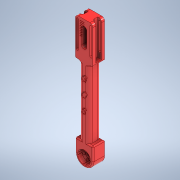
# Autodesk Inventor part: Eslabon1
Saved by Autodesk Inventor 2021 (Build 250183000, 183)
## iProperties
Created: 2022-10-26
Part Number: Eslabon1
Material: Generic
Document SubType Name: Modeling
Designer: USUARIO
Density: 1 g/cm^3
Appearance: Light Red
Mass: 84.0555 g
Surface Area: 248.63 cm^2
Volume: 84.0555 cm^3
Author: USUARIO
Autodesk Inventor part; units mm, degrees
ref_plane "YZ Plane" through (0, 0, 0) normal (1, 0, 0) x (0, 1, 0)
ref_plane "XZ Plane" through (0, 0, 0) normal (0, 1, 0) x (-1, 0, 0)
ref_plane "XY Plane" through (0, 0, 0) normal (0, 0, 1) x (1, 0, 0)
sketch "Sketch1" plane through (0, 0, 0) normal (0, 0, 1) x (1, 0, 0)
  line L0 (0, 0) -> (0, 190) construction
  line L1 (15, 0) -> (15, 190)
  line L2 (-15, 190) -> (-15, 0)
  arc A0 (-15, 0) -> (15, 0) centre (0, 0) ccw
  arc A1 (15, 190) -> (-15, 190) centre (0, 190) ccw
  line L3 (-15, 175) -> (15, 175)
  line L4 (15, 175) -> (15, 200)
  line L5 (10, 205) -> (-10, 205)
  line L6 (-15, 200) -> (-15, 175)
  line L7 (-15, 175) -> (15, 205) construction
  line L8 (15, 175) -> (-15, 205) construction
  arc A2 (-10, 205) -> (-15, 200) centre (-10, 200) ccw
  arc A3 (15, 200) -> (10, 205) centre (10, 200) ccw
  point P0 (0, 95)
  point P1 (0, 205)
  dimension "d0" = 190
  dimension "d1" = 30
  dimension "d48" = 5
  dimension "d49" = 30
  dimension "d50" = 30
  constraints: 20 end point, 8 point on circle, 8 tangent, 4 centre point, 4 point on line, 3 midpoint, 3 parallel, 1 equal radius, 1 horizontal, 1 perpendicular, 1 vertical
  measures "d0" distance of L0.start L0.end
  measures "d1" diameter of A1
  measures "d48" radius of A2
  measures "d49" distance between parallel lines of L6 L4
  measures "d50" distance between parallel lines of L3 L5
extrude "Extrusion1" add sketch "Sketch1" along normal blind 20
sketch "Sketch2" plane through (0, 0, 20) normal (0, 0, 1) x (1, 0, 0)
  arc A0 (15, 185) -> (-15, 185) centre (0, 185) ccw projected
  arc A1 (-15, 0) -> (15, 0) centre (0, 0) ccw projected
  circle A2 centre (0, 0) radius 11
  dimension "d4" = 22
  constraints: 1 centre point, 1 coincident
  measures "d4" diameter of A2
extrude "Extrusion2" cut sketch "Sketch2" against normal blind 7
sketch "Sketch3" plane through (0, 0, 0) normal (0, 0, -1) x (-1, 0, 0)
  circle A0 centre (0, 0) radius 11 projected
  circle A1 centre (0, 0) radius 11
  circle A2 centre (0, 0) radius 2
  circle A3 centre (0, 0) radius 8 construction
  arc A4 (15, 185) -> (-15, 185) centre (0, 185) ccw construction
  circle A5 centre (0, 8) radius 1.5
  line L0 (0, 0) -> (0, 12.8172) construction
  circle A6 centre (-8, 0) radius 1.5
  circle A7 centre (0, -8) radius 1.5
  circle A8 centre (8, 0) radius 1.5
  circle A9 centre (0, 0) radius 5
  dimension "d9" = 16
  dimension "d7" = 22
  dimension "d8" = 4
  dimension "d10" = 3
  dimension "d13" = 360
  dimension "d15" = 10
  constraints: 7 centre point, 4 coincident, 2 end point, 1 point on line, 1 vertical, 1 vertical alignment, 11 other
  measures "d7" diameter of A1
  measures "d8" diameter of A2
  measures "d10" diameter of A5
  measures "d15" diameter of A9
extrude "Extrusion4" cut sketch "Sketch3" against normal through all contours A5 | A6 | A7 | A8
sketch "Sketch4" plane through (0, 0, 13) normal (0, 0, 1) x (1, 0, 0)
  circle A0 centre (-8, 0) radius 1.5 projected
  circle A1 centre (0, 0) radius 2 construction
  circle A2 centre (0, 0) radius 8 construction
  line L0 (-5, 1.7321) -> (-5, -1.7321)
  line L1 (-5, -1.7321) -> (-8, -3.4641)
  line L2 (-8, -3.4641) -> (-11, -1.7321)
  line L3 (-11, -1.7321) -> (-11, 1.7321)
  line L4 (-11, 1.7321) -> (-8, 3.4641)
  line L5 (-8, 3.4641) -> (-5, 1.7321)
  line L6 (-3.4641, -8) -> (-1.7321, -5)
  line L7 (-1.7321, -5) -> (1.7321, -5)
  line L8 (1.7321, -5) -> (3.4641, -8)
  line L9 (3.4641, -8) -> (1.7321, -11)
  line L10 (1.7321, -11) -> (-1.7321, -11)
  line L11 (-1.7321, -11) -> (-3.4641, -8)
  line L12 (8, -3.4641) -> (5, -1.7321)
  line L13 (5, -1.7321) -> (5, 1.7321)
  line L14 (5, 1.7321) -> (8, 3.4641)
  line L15 (8, 3.4641) -> (11, 1.7321)
  line L16 (11, 1.7321) -> (11, -1.7321)
  line L17 (11, -1.7321) -> (8, -3.4641)
  line L18 (3.4641, 8) -> (1.7321, 5)
  line L19 (1.7321, 5) -> (-1.7321, 5)
  line L20 (-1.7321, 5) -> (-3.4641, 8)
  line L21 (-3.4641, 8) -> (-1.7321, 11)
  line L22 (-1.7321, 11) -> (1.7321, 11)
  line L23 (1.7321, 11) -> (3.4641, 8)
  dimension "d20" = 6
  dimension "d23" = 360
  constraints: 48 end point, 3 coincident, 1 horizontal alignment, 1 vertical, 64 other
  measures "d20" distance between parallel lines of L3 L0
extrude "Extrusion5" cut sketch "Sketch4" along normal blind 8.175 and the other way blind 3.5
extrude "Extrusion6" cut sketch "Sketch3" against normal blind 2 contours A0 | A2 | A9
extrude "Extrusion7" cut sketch "Sketch3" against normal through all contours A2
sketch "Sketch5" plane through (0, 0, 13) normal (0, 0, 1) x (1, 0, 0)
  circle A0 centre (0, 0) radius 2 projected
  circle A1 centre (0, 0) radius 4.5
  dimension "d33" = 9
  constraints: 1 centre point, 1 coincident
  measures "d33" diameter of A1
extrude "Extrusion8" cut sketch "Sketch5" against normal blind 3
sketch "Sketch9" plane through (0, 0, 20) normal (0, 0, 1) x (1, 0, 0)
  line L0 (-15, 200) -> (-15, 0) projected
  arc A0 (-15, 0) -> (15, 0) centre (0, 0) ccw projected
  line L1 (15, 0) -> (15, 200) projected
  arc A1 (15, 200) -> (10, 205) centre (10, 200) ccw projected
  line L2 (10, 205) -> (-10, 205) projected
  arc A2 (-10, 205) -> (-15, 200) centre (-10, 200) ccw projected
  line L3 (10.8485, 1.8195) -> (11, 1.7321) projected
  line L4 (11, 1.7321) -> (11, -1.7321) projected
  line L5 (11, -1.7321) -> (10.8485, -1.8195) projected
  arc A3 (1.8195, -10.8485) -> (10.8485, -1.8195) centre (0, 0) ccw projected
  line L6 (1.8195, -10.8485) -> (1.7321, -11) projected
  line L7 (1.7321, -11) -> (-1.7321, -11) projected
  line L8 (-1.7321, -11) -> (-1.8195, -10.8485) projected
  arc A4 (-10.8485, -1.8195) -> (-1.8195, -10.8485) centre (0, 0) ccw projected
  line L9 (-10.8485, -1.8195) -> (-11, -1.7321) projected
  line L10 (-11, -1.7321) -> (-11, 1.7321) projected
  line L11 (-11, 1.7321) -> (-10.8485, 1.8195) projected
  arc A5 (-1.8195, 10.8485) -> (-10.8485, 1.8195) centre (0, 0) ccw projected
  line L12 (-1.8195, 10.8485) -> (-1.7321, 11) projected
  line L13 (-1.7321, 11) -> (1.7321, 11) projected
  line L14 (1.7321, 11) -> (1.8195, 10.8485) projected
  arc A6 (10.8485, 1.8195) -> (1.8195, 10.8485) centre (0, 0) ccw projected
  line L15 (10, 205) -> (-10, 205) projected
  circle A7 centre (0, 0) radius 2 projected
  line L16 (0, 205) -> (0, 0) construction
  line L17 (0, 190) -> (0, 165) construction
  line L18 (-4.5, 190) -> (-4.5, 165)
  line L19 (4.5, 165) -> (4.5, 190)
  arc A8 (4.5, 190) -> (-4.5, 190) centre (0, 190) ccw
  arc A9 (-4.5, 165) -> (4.5, 165) centre (0, 165) ccw
  point P0 (0, 177.5)
  dimension "d51" = 25
  dimension "d52" = 9
  dimension "d53" = 190
  constraints: 10 end point, 4 point on circle, 4 tangent, 2 centre point, 2 midpoint, 2 point on line, 1 parallel, 1 vertical
  measures "d51" distance of L17.start L17.end
  measures "d52" diameter of A9
  measures "d53" distance of point (0, 0) L17.start
extrude "Extrusion11" cut sketch "Sketch9" against normal through all contours A8 L19 A9 L18
sketch "Sketch10" plane through (-10, 205, 0) normal (0, 1, 0) x (1, 0, 0)
  line L0 (14.5, -20) -> (5.5, -20) projected
  line L1 (5.5, -20) -> (14.5, -20) projected
  line L2 (-5, -20) -> (25, -20) projected
  line L3 (25, -20) -> (20, -20) projected
  line L4 (20, -20) -> (0, -20) projected
  line L5 (0, -20) -> (-5, -20) projected
  line L6 (20.8485, -20) -> (21, -20) projected
  line L7 (21, -20) -> (20.8485, -20) projected
  line L8 (20.8485, -20) -> (11.8195, -20) projected
  line L9 (11.8195, -20) -> (11.7321, -20) projected
  line L10 (11.7321, -20) -> (8.2679, -20) projected
  line L11 (8.2679, -20) -> (8.1805, -20) projected
  line L12 (8.1805, -20) -> (-0.8485, -20) projected
  line L13 (-0.8485, -20) -> (-1, -20) projected
  line L14 (-1, -20) -> (-0.8485, -20) projected
  line L15 (-0.8485, -20) -> (8.1805, -20) projected
  line L16 (8.1805, -20) -> (8.2679, -20) projected
  line L17 (8.2679, -20) -> (11.7321, -20) projected
  line L18 (11.7321, -20) -> (11.8195, -20) projected
  line L19 (11.8195, -20) -> (20.8485, -20) projected
  line L20 (25, 0) -> (25, -20) projected
  line L21 (25, 0) -> (25, -20) projected
  line L22 (14.5, 0) -> (5.5, 0) projected
  line L23 (5.5, 0) -> (14.5, 0) projected
  line L24 (-1, 0) -> (21, 0) projected
  line L25 (0, 0) -> (-5, 0) projected
  line L26 (20, 0) -> (0, 0) projected
  line L27 (25, 0) -> (20, 0) projected
  line L28 (-5, 0) -> (25, 0) projected
  line L29 (-5, 0) -> (-5, -20) projected
  line L30 (-5, 0) -> (-5, -20) projected
  line L31 (-5, 0) -> (-5, -20) projected
  line L32 (-5, -5) -> (2, -5)
  line L33 (2, -5) -> (2, -15)
  line L34 (2, -15) -> (-5, -15)
  line L35 (-5, -15) -> (-5, -5)
  line L36 (10, 0) -> (10, -20)
  line L37 (-5, -20) -> (25, -20) projected
  line L38 (25, -5) -> (18, -5)
  line L39 (18, -5) -> (18, -15)
  line L40 (18, -15) -> (25, -15)
  line L41 (25, -15) -> (25, -5)
  point P0 (-5, -15)
  dimension "d56" = 5
  dimension "d57" = 5
  dimension "d58" = 7
  constraints: 18 end point, 4 symmetric about line, 2 parallel, 1 horizontal, 1 perpendicular, 4 other
  measures "d56" distance between parallel lines of L28 L32
  measures "d57" distance between parallel lines of L2 L34
  measures "d58" distance of L33.end L34.end
extrude "Extrusion12" cut sketch "Sketch10" against normal blind 60 contours L40 L39 L38 L20 | L32 L33 L34 L29
sketch "Sketch11" plane through (0, 0, 0) normal (0, 0, -1) x (-1, 0, 0)
  arc A0 (-10, 205) -> (-15, 200) centre (-10, 200) ccw projected
  line L0 (-15, 145) -> (-15, 200) projected
  line L1 (-15, 145) -> (-8, 145) projected
  line L2 (-8, 205) -> (-8, 145) projected
  line L3 (-10, 205) -> (-8, 205) projected
  arc A1 (15, 200) -> (10, 205) centre (10, 200) ccw projected
  line L4 (8, 205) -> (10, 205) projected
  line L5 (8, 205) -> (8, 145) projected
  line L6 (8, 145) -> (15, 145) projected
  line L7 (15, 200) -> (15, 145) projected
  line L8 (-11.5, 145) -> (-11.5, 208.2052) construction
  line L9 (-11.5, 200) -> (-11.5, 155) construction
  line L10 (-13.2, 200) -> (-13.2, 155)
  line L11 (-9.8, 155) -> (-9.8, 200)
  arc A2 (-9.8, 200) -> (-13.2, 200) centre (-11.5, 200) ccw
  arc A3 (-13.2, 155) -> (-9.8, 155) centre (-11.5, 155) ccw
  arc A4 (-4.5, 165) -> (4.5, 165) centre (0, 165) ccw projected
  line L12 (4.5, 190) -> (4.5, 165) projected
  line L13 (-4.5, 165) -> (-4.5, 190) construction
  line L14 (-4.5, 177.5) -> (-11.5, 177.5) construction
  line L15 (-10, 205) -> (10, 205) projected
  line L16 (0, 205) -> (0, 150.8166) construction
  line L17 (13.2, 200) -> (13.2, 155)
  line L18 (9.8, 155) -> (9.8, 200)
  arc A5 (13.2, 200) -> (9.8, 200) centre (11.5, 200) ccw
  arc A6 (9.8, 155) -> (13.2, 155) centre (11.5, 155) ccw
  point P0 (0, 0)
  dimension "d61" = 3.4
  dimension "d62" = 45
  dimension "d73" = 23
  constraints: 18 end point, 8 point on circle, 6 symmetric about line, 4 centre point, 4 midpoint, 4 tangent, 2 point on line, 2 vertical, 1 horizontal, 1 parallel, 2 other
  measures "d61" diameter of A3
  measures "d62" distance of L10.start L10.end
  measures "d73" distance of A5.centre L9.start
extrude "Extrusion13" cut sketch "Sketch11" against normal through all contours A2 L11 A3 L10 | L17 A6 L18 A5
fillet "Fillet1" radius 4 2 edges at (8, 175, 15) (-8, 175, 15)
sketch "Sketch12" plane through (0, 0, 20) normal (0, 0, 1) x (1, 0, 0)
  line L0 (-18.3068, 122.2397) -> (15.3464, 122.2397) construction
  line L1 (15.3464, 122.2397) -> (15.3464, 18.2543) construction
  line L2 (15.3464, 18.2543) -> (-18.3068, 18.2543) construction
  line L3 (-18.3068, 18.2543) -> (-18.3068, 122.2397) construction
  line L4 (4.9339, 119.3269) -> (3.4605, 118.9967)
  spline S0 degree 2 poles (3.4605, 118.9967) (3.6299, 121.0289) (1.8856, 121.0289) knots 0 0 0 1 1 1
  spline S1 degree 2 poles (1.8856, 121.0289) (0.5647, 121.0289) (-0.5615, 119.9027) knots 0 0 0 1 1 1
  spline S2 degree 2 poles (-0.5615, 119.9027) (-1.603, 118.8612) (-2.2126, 117.0746) knots 0 0 0 1 1 1
  spline S3 degree 2 poles (-2.2126, 117.0746) (-2.907, 115.0085) (-2.4158, 113.9755) knots 0 0 0 1 1 1
  spline S4 degree 2 poles (-2.4158, 113.9755) (-2.0009, 113.1034) (-0.824, 113.1034) knots 0 0 0 1 1 1
  spline S5 degree 2 poles (-0.824, 113.1034) (0.3361, 113.1034) (1.3013, 114.0941) knots 0 0 0 1 1 1
  spline S6 degree 2 poles (1.3013, 114.0941) (2.0888, 114.9069) (2.5206, 116.0416) knots 0 0 0 1 1 1
  line L5 (2.5206, 116.0416) -> (-0.0534, 116.0416)
  line L6 (-0.0534, 116.0416) -> (0.353, 117.2355)
  line L7 (0.353, 117.2355) -> (4.2819, 117.2355)
  line L8 (4.2819, 117.2355) -> (2.5122, 112.0365)
  line L9 (2.5122, 112.0365) -> (1.4453, 112.0365)
  line L10 (1.4453, 112.0365) -> (1.8771, 113.5945)
  spline S7 degree 2 poles (1.8771, 113.5945) (1.3775, 112.7562) (0.4123, 112.2905) knots 0 0 0 1 1 1
  spline S8 degree 2 poles (0.4123, 112.2905) (-0.4345, 111.8841) (-1.332, 111.8841) knots 0 0 0 1 1 1
  spline S9 degree 2 poles (-1.332, 111.8841) (-3.3219, 111.8841) (-3.923, 113.4251) knots 0 0 0 1 1 1
  spline S10 degree 2 poles (-3.923, 113.4251) (-4.465, 114.8053) (-3.6944, 117.0577) knots 0 0 0 1 1 1
  spline S11 degree 2 poles (-3.6944, 117.0577) (-2.8307, 119.6148) (-0.9933, 121.0373) knots 0 0 0 1 1 1
  spline S12 degree 2 poles (-0.9933, 121.0373) (0.5562, 122.2397) (2.2836, 122.2397) knots 0 0 0 1 1 1
  spline S13 degree 2 poles (2.2836, 122.2397) (3.7654, 122.2397) (4.248, 121.4184) knots 0 0 0 1 1 1
  spline S14 degree 2 poles (4.248, 121.4184) (5.027, 120.6563) (4.9339, 119.3269) knots 0 0 0 1 1 1
  spline S15 degree 2 poles (2.1269, 98.052) (4.1168, 98.052) (4.5063, 96.5702) knots 0 0 0 1 1 1
  spline S16 degree 2 poles (4.5063, 96.5702) (5.2853, 95.1308) (4.5232, 92.8954) knots 0 0 0 1 1 1
  spline S17 degree 2 poles (4.5232, 92.8954) (3.651, 90.3298) (1.839, 88.8988) knots 0 0 0 1 1 1
  spline S18 degree 2 poles (1.839, 88.8988) (0.3149, 87.6964) (-1.3955, 87.6964) knots 0 0 0 1 1 1
  spline S19 degree 2 poles (-1.3955, 87.6964) (-3.3854, 87.6964) (-4.0035, 89.2459) knots 0 0 0 1 1 1
  spline S20 degree 2 poles (-4.0035, 89.2459) (-4.5454, 90.6261) (-3.7918, 92.8615) knots 0 0 0 1 1 1
  spline S21 degree 2 poles (-3.7918, 92.8615) (-2.9112, 95.4271) (-1.1076, 96.8497) knots 0 0 0 1 1 1
  spline S22 degree 2 poles (-1.1076, 96.8497) (0.4165, 98.052) (2.1269, 98.052) knots 0 0 0 1 1 1
  spline S23 degree 2 poles (1.712, 96.8412) (0.425, 96.8412) (-0.5742, 95.9352) knots 0 0 0 1 1 1
  spline S24 degree 2 poles (-0.5742, 95.9352) (-1.6834, 94.682) (-2.3015, 92.8869) knots 0 0 0 1 1 1
  spline S25 degree 2 poles (-2.3015, 92.8869) (-2.9959, 90.8293) (-2.5048, 89.7794) knots 0 0 0 1 1 1
  spline S26 degree 2 poles (-2.5048, 89.7794) (-2.0983, 88.9157) (-0.9806, 88.9157) knots 0 0 0 1 1 1
  spline S27 degree 2 poles (-0.9806, 88.9157) (0.3149, 88.9157) (1.314, 89.8387) knots 0 0 0 1 1 1
  spline S28 degree 2 poles (1.314, 89.8387) (2.4233, 91.0834) (3.0329, 92.8869) knots 0 0 0 1 1 1
  spline S29 degree 2 poles (3.0329, 92.8869) (3.7357, 94.9445) (3.2446, 95.986) knots 0 0 0 1 1 1
  spline S30 degree 2 poles (3.2446, 95.986) (2.8382, 96.8412) (1.712, 96.8412) knots 0 0 0 1 1 1
  line L11 (4.3708, 71.3326) -> (2.8551, 70.9431)
  spline S31 degree 2 poles (2.8551, 70.9431) (2.9398, 72.6705) (1.4749, 72.6705) knots 0 0 0 1 1 1
  spline S32 degree 2 poles (1.4749, 72.6705) (0.5604, 72.6705) (-0.0831, 72.2217) knots 0 0 0 1 1 1
  spline S33 degree 2 poles (-0.0831, 72.2217) (-0.625, 71.8407) (-0.8367, 71.231) knots 0 0 0 1 1 1
  spline S34 degree 2 poles (-0.8367, 71.231) (-1.0907, 70.4689) (-0.7689, 70.0964) knots 0 0 0 1 1 1
  spline S35 degree 2 poles (-0.7689, 70.0964) (-0.4641, 69.7492) (0.4842, 69.4952) knots 0 0 0 1 1 1
  line L12 (0.4842, 69.4952) -> (0.8568, 69.3766)
  spline S36 degree 2 poles (0.8568, 69.3766) (2.5418, 68.9025) (2.889, 67.9033) knots 0 0 0 1 1 1
  spline S37 degree 2 poles (2.889, 67.9033) (3.2446, 67.4884) (2.8805, 66.4131) knots 0 0 0 1 1 1
  spline S38 degree 2 poles (2.8805, 66.4131) (2.3979, 64.999) (0.8737, 64.1777) knots 0 0 0 1 1 1
  spline S39 degree 2 poles (0.8737, 64.1777) (-0.0661, 63.5087) (-1.5987, 63.5087) knots 0 0 0 1 1 1
  spline S40 degree 2 poles (-1.5987, 63.5087) (-3.0975, 63.5087) (-3.8003, 64.2369) knots 0 0 0 1 1 1
  spline S41 degree 2 poles (-3.8003, 64.2369) (-4.4353, 64.8889) (-4.3422, 66.1675) knots 0 0 0 1 1 1
  line L13 (-4.3422, 66.1675) -> (-2.818, 66.6247)
  spline S42 degree 2 poles (-2.818, 66.6247) (-2.9112, 65.5663) (-2.3693, 65.0159) knots 0 0 0 1 1 1
  spline S43 degree 2 poles (-2.3693, 65.0159) (-1.9798, 64.7026) (-1.2177, 64.7026) knots 0 0 0 1 1 1
  spline S44 degree 2 poles (-1.2177, 64.7026) (-0.1, 64.7026) (0.6028, 65.2107) knots 0 0 0 1 1 1
  spline S45 degree 2 poles (0.6028, 65.2107) (1.1616, 65.6086) (1.3902, 66.286) knots 0 0 0 1 1 1
  spline S46 degree 2 poles (1.3902, 66.286) (1.6527, 67.0566) (1.3394, 67.4207) knots 0 0 0 1 1 1
  spline S47 degree 2 poles (1.3394, 67.4207) (1.0262, 67.8102) (-0.0915, 68.1319) knots 0 0 0 1 1 1
  line L14 (-0.0915, 68.1319) -> (-0.4472, 68.2505)
  spline S48 degree 2 poles (-0.4472, 68.2505) (-1.9374, 68.6993) (-2.2761, 69.673) knots 0 0 0 1 1 1
  spline S49 degree 2 poles (-2.2761, 69.673) (-2.6402, 70.0879) (-2.2677, 71.1802) knots 0 0 0 1 1 1
  spline S50 degree 2 poles (-2.2677, 71.1802) (-1.8612, 72.391) (-0.6589, 73.1531) knots 0 0 0 1 1 1
  spline S51 degree 2 poles (-0.6589, 73.1531) (0.4588, 73.8644) (1.856, 73.8644) knots 0 0 0 1 1 1
  spline S52 degree 2 poles (1.856, 73.8644) (4.447, 73.8644) (4.3708, 71.3326) knots 0 0 0 1 1 1
  point P0 (0, 0)
  constraints: 2 other
extrude "Extrusion14" cut sketch "Sketch12" against normal blind 3
sketch "Sketch15" plane through (0, 0, 20) normal (0, 0, 1) x (1, 0, 0)
  line L0 (-9, 141.3) -> (9, 141.3)
  line L1 (9, 141.3) -> (9, 23)
  line L2 (9, 23) -> (-9, 23)
  line L3 (-9, 23) -> (-9, 141.3)
  line L4 (-15, 200) -> (-15, 0) projected
  line L5 (15, 0) -> (15, 200) projected
  arc A0 (9.8, 155) -> (13.2, 155) centre (11.5, 155) ccw projected
  line L6 (-1.7321, 11) -> (1.7321, 11) projected
  line L7 (-9, 141.3) -> (-15, 141.3)
  line L8 (-15, 145) -> (-15, 200) projected
  line L9 (9, 141.3) -> (15, 141.3)
  line L10 (15, 0) -> (15, 200) projected
  line L11 (9, 23) -> (15, 23)
  line L12 (-9, 23) -> (-15, 23)
  point P0 (0, 0)
  point P1 (-15, 141.3)
  point P2 (15, 141.3)
  dimension "d74" = 6
  dimension "d75" = 6
  dimension "d76" = 12
  dimension "d77" = 12
  constraints: 16 end point, 6 point on line, 2 horizontal, 2 parallel, 2 perpendicular
  measures "d74" distance between parallel lines of L4 L3
  measures "d75" distance between parallel lines of L5 L1
  measures "d76" distance edge to line of A0 L0
  measures "d77" distance between parallel lines of L6 L2
extrude "Extrusion15" cut sketch "Sketch15" against normal through all contours L3 L12 L4 L7 | L9 L5 L11 L1
fillet "Fillet2" radius 6 4 edges at (9, 82.15, 20) (9, 82.15, 0) (-9, 82.15, 20) (-9, 82.15, 0)
fillet "Fillet3" radius 4 6 edges at (9, 141.3, 10) (7.2426, 141.3, 18.2426) (-9, 141.3, 10) (-7.2426, 141.3, 18.2426) (7.2426, 141.3, 1.7574) (-7.2426, 141.3, 1.7574)
fillet "Fillet4" radius 2 2 edges at (-15, 141.3, 10) (15, 141.3, 10)
fillet "Fillet5" radius 2 9 edges at (15, 23, 10) (9, 23, 20) (9, 23, 0) (-9, 23, 20) (-15, 23, 10) (-9, 23, 0) (0, -15, 20) (15, 11.5, 20) (-15, 11.5, 20)
sketch "Sketch16" plane through (0, 0, 20) normal (0, 0, 1) x (1, 0, 0)
  line L0 (15, 143.3) -> (15, 200) projected
  arc A0 (15, 200) -> (10, 205) centre (10, 200) ccw projected
  line L1 (10, 205) -> (-10, 205) projected
  arc A1 (-10, 205) -> (-15, 200) centre (-10, 200) ccw projected
  line L2 (-15, 200) -> (-15, 143.3) projected
  line L3 (-13, 21) -> (-3, 21) projected
  line L4 (-13, 0) -> (-13, 21) projected
  arc A2 (-13, 0) -> (13, 0) centre (0, 0) ccw projected
  line L5 (13, 21) -> (13, 0) projected
  line L6 (3, 21) -> (13, 21) projected
  line L7 (10.8485, 1.8195) -> (11, 1.7321) projected
  line L8 (11, 1.7321) -> (11, -1.7321) projected
  line L9 (11, -1.7321) -> (10.8485, -1.8195) projected
  arc A3 (1.8195, -10.8485) -> (10.8485, -1.8195) centre (0, 0) ccw projected
  line L10 (1.8195, -10.8485) -> (1.7321, -11) projected
  line L11 (1.7321, -11) -> (-1.7321, -11) projected
  line L12 (-1.7321, -11) -> (-1.8195, -10.8485) projected
  arc A4 (-10.8485, -1.8195) -> (-1.8195, -10.8485) centre (0, 0) ccw projected
  line L13 (-10.8485, -1.8195) -> (-11, -1.7321) projected
  line L14 (-11, -1.7321) -> (-11, 1.7321) projected
  line L15 (-11, 1.7321) -> (-10.8485, 1.8195) projected
  arc A5 (-1.8195, 10.8485) -> (-10.8485, 1.8195) centre (0, 0) ccw projected
  line L16 (-1.8195, 10.8485) -> (-1.7321, 11) projected
  line L17 (-1.7321, 11) -> (1.7321, 11) projected
  line L18 (1.7321, 11) -> (1.8195, 10.8485) projected
  arc A6 (10.8485, 1.8195) -> (1.8195, 10.8485) centre (0, 0) ccw projected
  line L19 (4.5, 190) -> (4.5, 165) projected
  arc A7 (-4.5, 165) -> (4.5, 165) centre (0, 165) ccw projected
  line L20 (-4.5, 165) -> (-4.5, 190) projected
  arc A8 (4.5, 190) -> (-4.5, 190) centre (0, 190) ccw projected
  line L21 (9.8, 155) -> (9.8, 200) projected
  arc A9 (13.2, 200) -> (9.8, 200) centre (11.5, 200) ccw projected
  line L22 (13.2, 200) -> (13.2, 155) projected
  arc A10 (9.8, 155) -> (13.2, 155) centre (11.5, 155) ccw projected
  arc A11 (-9.8, 200) -> (-13.2, 200) centre (-11.5, 200) ccw projected
  line L23 (-9.8, 200) -> (-9.8, 155) projected
  arc A12 (-13.2, 155) -> (-9.8, 155) centre (-11.5, 155) ccw projected
  line L24 (-13.2, 155) -> (-13.2, 200) projected
  line L25 (3, 70.9803) -> (2.8551, 70.9431) projected
  line L26 (0.4842, 69.4952) -> (0.8568, 69.3766) projected
  line L27 (-3, 66.5702) -> (-2.818, 66.6247) projected
  line L28 (-0.0915, 68.1319) -> (-0.4472, 68.2505) projected
  line L29 (2.5206, 116.0416) -> (-0.0534, 116.0416) projected
  line L30 (-0.0534, 116.0416) -> (0.353, 117.2355) projected
  line L31 (0.353, 117.2355) -> (3, 117.2355) projected
  line L32 (3, 113.4696) -> (2.5122, 112.0365) projected
  line L33 (2.5122, 112.0365) -> (1.4453, 112.0365) projected
  line L34 (1.4453, 112.0365) -> (1.8771, 113.5945) projected
  line L35 (-0.25, 200) -> (-7.25, 200) construction
  line L36 (-0.25, 200.25) -> (-7.25, 200.25)
  line L37 (-7.25, 199.75) -> (-0.25, 199.75)
  arc A13 (-0.25, 199.75) -> (-0.25, 200.25) centre (-0.25, 200) ccw
  arc A14 (-7.25, 200.25) -> (-7.25, 199.75) centre (-7.25, 200) ccw
  line L38 (0, -59.2071) -> (0, 250.2426) projected
  line L39 (-0.25, 195.25) -> (-7.25, 195.25)
  arc A15 (-7.25, 195.25) -> (-7.25, 194.75) centre (-7.25, 195) ccw
  line L40 (-7.25, 194.75) -> (-0.25, 194.75)
  arc A16 (-0.25, 194.75) -> (-0.25, 195.25) centre (-0.25, 195) ccw
  line L41 (-0.25, 190.25) -> (-7.25, 190.25)
  arc A17 (-7.25, 190.25) -> (-7.25, 189.75) centre (-7.25, 190) ccw
  line L42 (-7.25, 189.75) -> (-0.25, 189.75)
  arc A18 (-0.25, 189.75) -> (-0.25, 190.25) centre (-0.25, 190) ccw
  line L43 (-0.25, 185.25) -> (-7.25, 185.25)
  arc A19 (-7.25, 185.25) -> (-7.25, 184.75) centre (-7.25, 185) ccw
  line L44 (-7.25, 184.75) -> (-0.25, 184.75)
  arc A20 (-0.25, 184.75) -> (-0.25, 185.25) centre (-0.25, 185) ccw
  line L45 (-0.25, 180.25) -> (-7.25, 180.25)
  arc A21 (-7.25, 180.25) -> (-7.25, 179.75) centre (-7.25, 180) ccw
  line L46 (-7.25, 179.75) -> (-0.25, 179.75)
  arc A22 (-0.25, 179.75) -> (-0.25, 180.25) centre (-0.25, 180) ccw
  line L47 (-0.25, 197.5) -> (-7.25, 197.5) construction
  line L48 (-0.25, 197.75) -> (-7.25, 197.75)
  line L49 (-7.25, 197.25) -> (-0.25, 197.25)
  arc A23 (-0.25, 197.25) -> (-0.25, 197.75) centre (-0.25, 197.5) ccw
  arc A24 (-7.25, 197.75) -> (-7.25, 197.25) centre (-7.25, 197.5) ccw
  line L50 (-0.25, 192.75) -> (-7.25, 192.75)
  arc A25 (-7.25, 192.75) -> (-7.25, 192.25) centre (-7.25, 192.5) ccw
  line L51 (-7.25, 192.25) -> (-0.25, 192.25)
  arc A26 (-0.25, 192.25) -> (-0.25, 192.75) centre (-0.25, 192.5) ccw
  line L52 (-0.25, 187.75) -> (-7.25, 187.75)
  arc A27 (-7.25, 187.75) -> (-7.25, 187.25) centre (-7.25, 187.5) ccw
  line L53 (-7.25, 187.25) -> (-0.25, 187.25)
  arc A28 (-0.25, 187.25) -> (-0.25, 187.75) centre (-0.25, 187.5) ccw
  line L54 (-0.25, 182.75) -> (-7.25, 182.75)
  arc A29 (-7.25, 182.75) -> (-7.25, 182.25) centre (-7.25, 182.5) ccw
  line L55 (-7.25, 182.25) -> (-0.25, 182.25)
  arc A30 (-0.25, 182.25) -> (-0.25, 182.75) centre (-0.25, 182.5) ccw
  line L56 (-0.25, 177.75) -> (-7.25, 177.75)
  arc A31 (-7.25, 177.75) -> (-7.25, 177.25) centre (-7.25, 177.5) ccw
  line L57 (-7.25, 177.25) -> (-0.25, 177.25)
  arc A32 (-0.25, 177.25) -> (-0.25, 177.75) centre (-0.25, 177.5) ccw
  arc A33 (13, 141.3) -> (15, 143.3) centre (13, 143.3) ccw projected
  arc A34 (-15, 143.3) -> (-13, 141.3) centre (-13, 143.3) ccw projected
  line L58 (3, 120.6822) -> (3, 117.2355) projected
  line L59 (3, 70.9803) -> (3, 67.7172) projected
  line L60 (3, 66.8282) -> (3, 21) projected
  line L61 (-3, 21) -> (-3, 63.7265) projected
  line L62 (-3, 66.5702) -> (-3, 88.0592) projected
  line L63 (3, 90.049) -> (3, 73.7011) projected
  line L64 (-3, 94.6277) -> (-3, 112.2846) projected
  line L65 (3, 113.4696) -> (3, 97.9644) projected
  line L66 (-13, 141.3) -> (-11, 141.3) projected
  line L67 (-3, 118.6555) -> (-3, 137.3) projected
  line L68 (3, 137.3) -> (3, 122.1818) projected
  line L69 (11, 141.3) -> (13, 141.3) projected
  point P0 (-3.75, 200)
  point P1 (-3.75, 197.5)
  point P2 (-3.8971, 192.25)
  point P3 (-3.562, 192.75)
  point P4 (-4.5, 189.75)
  point P5 (-4.4931, 190.25)
  point P6 (-4.5, 187.25)
  point P7 (-4.5, 187.75)
  point P8 (-4.5, 184.75)
  point P9 (-4.5, 185.25)
  point P10 (-4.5, 182.25)
  point P11 (-4.5, 182.75)
  point P12 (-4.5, 179.75)
  point P13 (-4.5, 180.25)
  point P14 (-4.5, 177.25)
  point P15 (-4.5, 177.75)
  dimension "d84" = 7
  dimension "d85" = 0.5
  dimension "d86" = 10
  dimension "d89" = 5
  dimension "d94" = 7
  dimension "d95" = 0.5
  dimension "d96" = 7.5
  dimension "d99" = 5
  constraints: 48 end point, 40 point on circle, 20 centre point, 10 tangent, 2 midpoint, 2 parallel, 2 vertical, 1 horizontal, 1 perpendicular, 123 other
  measures "d84" distance of L35.start L35.end
  measures "d85" diameter of A14
  measures "d86" distance from line of A8.centre L35
  measures "d89" distance of L36.start L39.start
  measures "d94" distance of L47.start L47.end
  measures "d95" diameter of A24
  measures "d96" distance from line of A8.centre L47
  measures "d99" distance of L48.start L50.start
extrude "Extrusion16" cut sketch "Sketch16" against normal blind 1 contours A8 L51 A25 L50 | L57 A31 L56 L20 | A8 L20 L42 A17 L41 | L46 A21 L45 L20 | L53 A27 L52 L20 | L55 A29 L54 L20 | L44 A19 L43 L20 | A13 L37 A14 L36 | A16 L40 A15 L39 | A23 L49 A24 L48
equation "\"d0\" = L1"
equation "\"d1\" = B1"
equation "\"d49\" = B1"
equation "\"d50\" = d49"
equation "\"d2\" = H1"
equation "\"d4\" = DER"
equation "\"d5\" = HR"
equation "\"d7\" = DER"
equation "\"d8\" = DEM"
equation "\"d53\" = Dmax"
equation "\"d57\" = d56"
equation "\"d74\" = RC"
equation "\"d75\" = RC"
equation "\"d76\" = 2 * RC"
equation "\"d77\" = 2 * RC"
equation "\"d80\" = RC"
equation "\"d81\" = 0.666667 * RC"
equation "\"L1\" = 190"
equation "\"B1\" = 30"
equation "\"H1\" = 20"
equation "\"DER\" = 22"
equation "\"DIR\" = 8"
equation "\"HR\" = 7"
equation "\"DEM\" = 4"
equation "\"Dmax\" = 190"
equation "\"Bsm\" = 22.5"
equation "\"Dmarc\" = 17.5"
equation "\"Hsm\" = 12"
equation "\"Dsc\" = 5"
equation "\"Lsm\" = 21"
equation "\"RC\" = 6"
equation "\"TB\" = 3"
equation "\"HSE\" = 25"
equation "\"PB\" = 25"
equation "\"LMaSP\" = 46.5"
body "Solid1"
